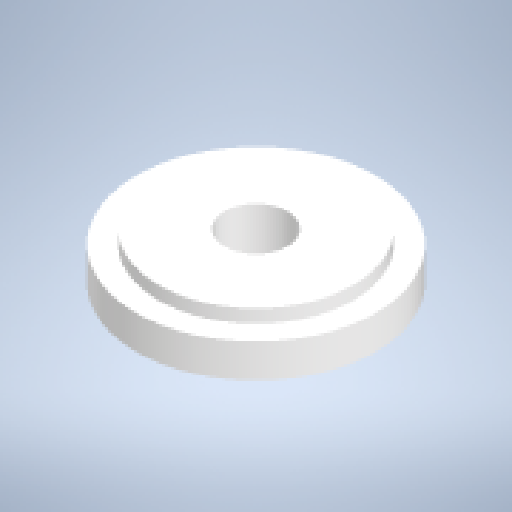
# Autodesk Inventor part: 035
Saved by Autodesk Inventor 2023 (Build 270158000, 158)
## iProperties
Created: 2022-04-25
Part Number: 035
Material: Polyethylene, High Density
Document SubType Name: Modeling
Designer: vmiguel
Density: 0.952 g/cm^3
Appearance: Smooth - White
Author: vmiguel
Autodesk Inventor part; units mm, degrees
ref_plane "YZ Plane" through (0, 0, 0) normal (1, 0, 0) x (0, 1, 0)
ref_plane "XZ Plane" through (0, 0, 0) normal (0, 1, 0) x (-1, 0, 0)
ref_plane "XY Plane" through (0, 0, 0) normal (0, 0, 1) x (1, 0, 0)
sketch "Sketch1" plane through (0, 0, 0) normal (0, 0, 1) x (1, 0, 0)
  line L0 (0, 0) -> (0, 3.0949)
  line L1 (3.5, 0) -> (3.5, 3.8)
  line L2 (3.5, 3.8) -> (13.5, 3.8)
  line L3 (13.5, 3.8) -> (13.5, 0)
  line L4 (13.5, 0) -> (12, 0)
  line L5 (12, 0) -> (12, 1.23)
  line L6 (12, 1.23) -> (10, 1.23)
  line L7 (10, 1.23) -> (10, 0)
  line L8 (10, 0) -> (3.5, 0)
  line L9 (11, 3.8) -> (11, 5.3)
  line L10 (11, 5.3) -> (3.5, 5.3)
  line L11 (3.5, 5.3) -> (3.5, 3.8)
  dimension "d0" = 7
  dimension "d1" = 27
  dimension "d2" = 2
  dimension "d3" = 1.23
  dimension "d4" = 3.8
  dimension "d5" = 20
  dimension "d7" = 22
  dimension "d8" = 1.5
  constraints: 24 end point, 8 perpendicular, 3 vertical, 2 point on line, 1 collinear, 1 horizontal alignment
  measures "d0" diameter of L1 L0
  measures "d1" diameter of L3 L0
  measures "d2" distance of L5.end L6.end
  measures "d3" distance of L4.end L5.end
  measures "d4" distance of L2.end L3.end
  measures "d5" diameter of L7 L0
  measures "d7" diameter of L9 L0
  measures "d8" distance of L9.start L9.end
revolve "Revolution1" add sketch "Sketch1" angle 360 about axis through (0, 0, 0) along (0, 1, 0)
body "Solid1"
